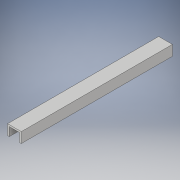
# Autodesk Inventor part: case
Saved by Autodesk Inventor 2017 (Build 210142000, 142)
## iProperties
Created: 2017-10-11
Part Number: case
Material: Generic
Document SubType Name: Modeling
Designer: Kenneth
Density: 1 g/cm^3
Appearance: Default
Author: Kenneth
Autodesk Inventor part; units mm, degrees
ref_plane "YZ Plane" through (0, 0, 0) normal (1, 0, 0) x (0, 1, 0)
ref_plane "XZ Plane" through (0, 0, 0) normal (0, 1, 0) x (-1, 0, 0)
ref_plane "XY Plane" through (0, 0, 0) normal (0, 0, 1) x (1, 0, 0)
sketch "Sketch1" plane through (0, 0, 0) normal (0, 0, 1) x (1, 0, 0)
  line L0 (12.7, -9.525) -> (12.7, 9.525)
  line L1 (12.7, 9.525) -> (-12.7, 9.525)
  line L2 (-12.7, 9.525) -> (-12.7, -9.525)
  line L3 (-12.7, -9.525) -> (12.7, 9.525) construction
  line L4 (12.7, -9.525) -> (-12.7, 9.525) construction
  line L5 (9.525, -6.35) -> (9.525, 6.35)
  line L6 (9.525, 6.35) -> (-9.525, 6.35)
  line L7 (-9.525, 6.35) -> (-9.525, -6.35)
  line L8 (-9.525, -6.35) -> (9.525, 6.35) construction
  line L9 (9.525, -6.35) -> (-9.525, 6.35) construction
  line L10 (-9.525, -6.35) -> (-9.525, -9.525)
  line L11 (-9.525, -9.525) -> (-12.7, -9.525)
  line L12 (9.525, -6.35) -> (9.525, -9.525)
  line L13 (9.525, -9.525) -> (12.7, -9.525)
  point P0 (0, 0)
  dimension "d0" = 25.4
  dimension "d1" = 19.05
  dimension "d4" = 19.05
  dimension "d5" = 12.7
  dimension "d6" = 90
  constraints: 28 end point, 4 midpoint, 3 parallel, 1 perpendicular, 1 vertical
  measures "d0" distance of L0.end L1.end
  measures "d1" distance of L0.start L0.end
  measures "d4" distance of L5.end L6.end
  measures "d5" distance of L5.start L5.end
  measures "d6" angle of L10 L11
extrude "Extrusion2" add sketch "Sketch1" along normal blind 279.4
body "Solid2"
